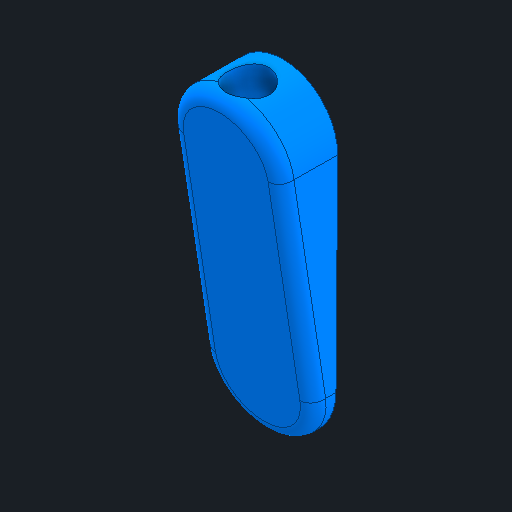
# Autodesk Inventor part: shaft_outlet
Saved by Autodesk Inventor 2023 (Build 270158030, 158C)
## iProperties
Created: 2022-03-28
Part Number: shaft_outlet
Material: Generic
Document SubType Name: Modeling
Designer: kardo
Density: 1 g/cm^3
Appearance: Blue Plastic
Author: kardo
Autodesk Inventor part; units mm, degrees
ref_plane "YZ Plane" through (0, 0, 0) normal (1, 0, 0) x (0, 1, 0)
ref_plane "XZ Plane" through (0, 0, 0) normal (0, 1, 0) x (-1, 0, 0)
ref_plane "XY Plane" through (0, 0, 0) normal (0, 0, 1) x (1, 0, 0)
derived "stencil_frame.ipt"
sketch "sk_drivetrain_profile" plane through (6, 0, 0) normal (1, 0, 0) x (0, 1, 0)
  line L0 (-547.3485, 0) -> (393.091, 0) construction
  line L1 (-363, 4592.9714) -> (-363, -1605.7041) construction
  line L2 (0, 4592.9714) -> (0, -1605.7041) construction
  line L3 (-140.2591, 52.979) -> (-133.4853, 25.8107)
  line L4 (-388, 0) -> (-343.0839, 2.7472)
  line L5 (-136.8722, 39.3948) -> (-222.489, 18.0482)
  line L6 (-307.9329, 4.8971) -> (-264.6067, 7.5471) construction
  line L7 (-264.6067, 7.5471) -> (-222.489, 18.0482) construction
  line L8 (-133.4853, 25.8107) -> (-133.4853, 20.8107) construction
  line L9 (-343.0839, 2.7472) -> (-307.9329, 4.8971)
  line L10 (-1229.7832, 4422.8213) -> (280.3081, -1633.8241) construction
  spline S0 degree 2 poles (-307.9329, 4.8971) (-264.6067, 7.5471) (-222.489, 18.0482) knots 1 1 1 2 2 2
  line L11 (-223.0651, 20.3587) -> (-137.4483, 41.7054) construction
  line L12 (-136.2962, 37.0843) -> (-221.913, 15.7377) construction
  line L13 (-223.0651, 20.3587) -> (-221.913, 15.7377) construction
  line L14 (0, 18.496) -> (-254.1001, 20.6178) construction
  line L15 (-55.3282, 20.1581) -> (-309.4681, 22.2802) construction
  point P0 (0, 0)
  point P1 (-213.541, 20.2792)
  point P2 (-204.017, 20.1996)
  point P3 (-199.3598, 21.3608)
sketch "sk_prop_shaft_cut" plane through (6, 0, 18.496) normal (0, 0.0083502, 0.9999651) x (0, -0.9999651, 0.0083502)
  line L0 (223.0729, -4.3812) -> (199.3768, -4.3812)
  line L1 (223.0729, 4.3812) -> (199.3768, 4.3812)
  arc A0 (199.3768, 4.3812) -> (199.3768, -4.3812) centre (199.3768, 0) ccw
  arc A1 (223.0729, -4.3812) -> (223.0729, 4.3812) centre (223.0729, 0) ccw
  point P0 (-0.1544, -6)
  point P1 (213.5485, 0)
  point P2 (204.0241, 0)
ref_plane "plane_motor_mount" through (0, -127.05, 0) normal (0, 0.9702957, 0.2419219) x (-1, 0, 0)
derived "parameters_powertrain.ipt"
derived "parameters_frame.ipt"
extrude "lower_plate" add sketch "sk_prop_shaft_cut" along normal blind 1.2
sketch "sk_upper_plate" plane through (6, -223.0551, 21.5587) normal (0, 0.0083502, 0.9999651) x (1, 0, 0)
  line L0 (-4.3813, 23.6961) -> (-4.3813, 0) projected
  arc A0 (-4.3813, 0) -> (4.3812, 0) centre (0, 0) ccw projected
  line L1 (4.3812, 0) -> (4.3812, 23.6961) projected
  arc A1 (4.3812, 23.6961) -> (-4.3813, 23.6961) centre (0, 23.6961) ccw projected
  line L2 (-6.3812, 0) -> (-6.3813, 23.6961)
  arc A2 (6.3812, 23.6961) -> (-6.3813, 23.6961) centre (0, 23.6961) ccw
  line L3 (6.3812, 23.6961) -> (6.3812, 0)
  arc A3 (-6.3812, 0) -> (6.3812, 0) centre (0, 0) ccw
  point P0 (-6, 223.2273)
  dimension "d6" = 2
  constraints: 4 end point, 4 point on circle, 2 centre point, 3 other
  measures "d6" distance between parallel lines of L2 L0
extrude "upper_plate" add sketch "sk_upper_plate" along normal blind 7.62 contours A1 L1 A0 L0 | L2 A2 L3 A3
sketch "sk_trim" plane through (12.3813, -223.0551, 21.5587) normal (1, 0, 0) x (0, -0.0083502, -0.9999651)
  line L0 (-1.6669, -6.3813) -> (-7.62, 30.0773)
  line L1 (0, 0) -> (0, -6.3812) projected
  line L2 (-7.62, 30.0773) -> (-7.62, 23.6961) projected
  line L3 (0, -6.3812) -> (-1.6669, -6.3813)
  line L4 (-1.6669, -6.3813) -> (-7.62, -6.3813)
  line L5 (-7.62, -6.3813) -> (-7.62, 23.6961)
  dimension "d16" = 1.6669
  constraints: 8 end point, 2 collinear, 1 perpendicular
  measures "d16" distance of L1.end L0.start
extrude "trim" cut sketch "sk_trim" against normal through all
sketch "sk_drill" plane through (0, -127.05, 0) normal (0, 0.9702957, 0.2419219) x (-1, 0, 0)
  circle A0 centre (-6, 40.6009) radius 2.3813
  point P0 (0, -30.7362)
  dimension "d9" = 4.7625
  constraints: 1 centre point, 1 coincident
  measures "d9" diameter of A0
extrude "drill" cut sketch "sk_drill" along normal through all both and the other way through all
fillet "Fillet1" radius 1.5 6 edges at (10.5122, -227.5507, 23.5683) (1.4878, -227.5507, 23.5683) (-0.3812, -211.1687, 26.103) (10.5122, -194.7867, 28.6377) (1.4878, -194.7867, 28.6377) (12.3812, -211.1687, 26.103)
equation "\"d4\" = shell_thickness"
equation "\"d7\" = 1.6 * prop_shaft_od"
equation "\"d16\" = 0.35 * prop_shaft_od"
equation "\"d9\" = prop_shaft_od"
equation "\"shell_thickness\" = 1.2"
equation "\"prop_shaft_od\" = 4.7625"
body "Solid1"
